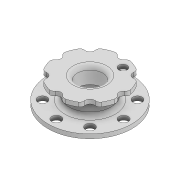
# Autodesk Inventor part: Pully_smlaller
Saved by Autodesk Inventor 2021 (Build 250183000, 183)
## iProperties
Created: 2022-09-22
Part Number: Pully_smlaller
Material: Generic
Document SubType Name: Modeling
Designer: ereg140
Density: 1 g/cm^3
Appearance: Default
Author: ereg140
Autodesk Inventor part; units mm, degrees
ref_plane "YZ Plane" through (0, 0, 0) normal (1, 0, 0) x (0, 1, 0)
ref_plane "XZ Plane" through (0, 0, 0) normal (0, 1, 0) x (-1, 0, 0)
ref_plane "XY Plane" through (0, 0, 0) normal (0, 0, 1) x (1, 0, 0)
sketch "Sketch1" plane through (0, 0, 0) normal (0, 1, 0) x (-1, 0, 0)
  circle A0 centre (0, 0) radius 12.0717
  line L0 (6, 10.475) -> (-6, 10.475)
  line L1 (9.5, 7.4482) -> (-9.5, 7.4482)
  dimension "d20" = 12
  dimension "d23" = 19
  dimension "d24" = 10.475
  constraints: 4 end point, 4 point on circle, 2 horizontal, 1 centre point, 1 coincident
  measures "d20" distance of L0.start L0.end
  measures "d23" distance of L1.start L1.end
  measures "d24" distance from line of point (0, 0) L0
extrude "Extrusion1" add sketch "Sketch1" along normal blind 3.8
sketch "Sketch2" plane through (0, 3.8, 0) normal (0, 1, 0) x (1, 0, 0)
  circle A0 centre (0, 0) radius 8 construction
  circle A1 centre (-8, 0) radius 1.1
  circle A2 centre (-5.6569, -5.6569) radius 1.1
  circle A3 centre (0, -8) radius 1.1
  circle A4 centre (5.6569, -5.6569) radius 1.1
  circle A5 centre (8, 0) radius 1.1
  circle A6 centre (5.6569, 5.6569) radius 1.1
  circle A7 centre (0, 8) radius 1.1
  circle A8 centre (-5.6569, 5.6569) radius 1.1
  circle A9 centre (0, 0) radius 5.5
  dimension "d3" = 16
  dimension "d4" = 2.2
  dimension "d7" = 360
  dimension "d9" = 11
  constraints: 9 centre point, 2 coincident, 2 horizontal alignment, 19 other
  measures "d4" diameter of A1
  measures "d9" diameter of A9
extrude "Extrusion2" cut sketch "Sketch2" against normal through all
sketch "Sketch3" plane through (0, 0, 0) normal (1, 0, 0) x (0, 1, 0)
  point P0 (0, 0)
sketch "Sketch4" plane through (0, 0, 0) normal (1, 0, 0) x (0, 1, 0)
  line L0 (3.8, 5.5) -> (0, 5.5) construction
  line L1 (0, 5.5) -> (0, 6.9) construction
  line L2 (0, 6.9) -> (3.8, 6.9) construction
  line L3 (3.8, 6.9) -> (3.8, 5.5) construction
  line L4 (0, -5.5) -> (3.8, -5.5) construction
  line L5 (3.8, -5.5) -> (3.8, -6.9) construction
  line L6 (3.8, -6.9) -> (0, -6.9) construction
  line L7 (0, -6.9) -> (0, -5.5) construction
  line L8 (0, 12.0717) -> (3.8, 12.0717) construction
  line L9 (3.8, 12.0717) -> (3.8, 9.1) construction
  line L10 (3.8, 9.1) -> (0, 9.1) construction
  line L11 (0, 9.1) -> (0, 12.0717) construction
  line L12 (3.8, -12.0717) -> (0, -12.0717) construction
  line L13 (0, -12.0717) -> (0, -9.1) construction
  line L14 (0, -9.1) -> (3.8, -9.1) construction
  line L15 (3.8, -9.1) -> (3.8, -12.0717) construction
  line L16 (0.6, -12.0717) -> (3.2, -12.0717)
  line L17 (3.2, -12.0717) -> (3.2, -9.5)
  line L18 (3.2, -9.5) -> (0.6, -9.5)
  line L19 (0.6, -9.5) -> (0.6, -12.0717)
  line L20 (-0.76, 0) -> (4.56, 0) projected
  point P0 (0, 0)
  point P1 (1.9, -12.0717)
  dimension "d12" = 0.6
  dimension "d15" = 9.5
  constraints: 8 end point, 2 midpoint, 2 parallel, 1 horizontal, 1 perpendicular
  measures "d12" distance between parallel lines of L13 L19
  measures "d15" distance from line of point (0, 0) L18
revolve "Revolution1" cut sketch "Sketch4" angle 360 about axis through (0, -10, 0) along (0, 1, 0)
sketch "Sketch5" plane through (0, 3.2, 0) normal (0, -1, 0) x (1, 0, 0)
  circle A0 centre (0, -10.1) radius 0.6
  circle A1 centre (0, 0) radius 9.5 construction
  circle A2 centre (0, 0) radius 12.0717 construction
  circle A3 centre (-8, 0) radius 1.1 construction
  circle A4 centre (8, 0) radius 1.1 construction
  circle A5 centre (5.6569, 5.6569) radius 1.1 construction
  circle A6 centre (-5.6569, -5.6569) radius 1.1 construction
  circle A7 centre (-5.6569, 5.6569) radius 1.1 construction
  circle A8 centre (5.6569, -5.6569) radius 1.1 construction
  circle A9 centre (0, 8) radius 1.1 construction
  circle A10 centre (0, -8) radius 1.1 construction
  circle A11 centre (0, 0) radius 5.5 construction
  dimension "d17" = 1.2
  constraints: 1 centre point, 1 tangent, 1 vertical alignment
  measures "d17" diameter of A0
extrude "Extrusion3" cut sketch "Sketch5" against normal up to surface (0.6 mm away)
sketch "Sketch6" plane through (0, 3.8, 0) normal (0, 1, 0) x (1, 0, 0)
  circle A0 centre (0, 0) radius 12.0717 projected
extrude "Extrusion4" cut sketch "Sketch6" against normal up to surface (3.2 mm away)
sketch "Sketch7" plane through (0, 0.6, 0) normal (0, 1, 0) x (1, 0, 0)
  circle A0 centre (0, 0) radius 5.5 projected
  circle A1 centre (0, 8) radius 1.1 projected
  circle A2 centre (0, -8) radius 1.1 projected
  circle A3 centre (5.6569, 5.6569) radius 1.1 projected
  circle A4 centre (-5.6569, -5.6569) radius 1.1 projected
  circle A5 centre (-5.6569, 5.6569) radius 1.1 projected
  circle A6 centre (5.6569, -5.6569) radius 1.1 projected
  circle A7 centre (8, 0) radius 1.1 projected
  circle A8 centre (-8, 0) radius 1.1 projected
  circle A9 centre (0, 0) radius 12.0717 projected
extrude "Extrusion5" add sketch "Sketch7" along normal blind 0.4
sketch "Sketch9" plane through (0, 0, 0) normal (0, -1, 0) x (1, 0, 0)
  circle A0 centre (0, 0) radius 4.25
  circle A1 centre (0, 0) radius 5.5 projected
  dimension "d29" = 8.5
  constraints: 1 centre point, 1 coincident
  measures "d29" diameter of A0
extrude "Extrusion6" add sketch "Sketch9" against normal up to surface (1 mm away)
sketch "Sketch10" plane through (0, 1, 0) normal (0, 1, 0) x (1, 0, 0)
  circle A0 centre (0, 0) radius 10
  circle A1 centre (0, 0) radius 12.0717 projected
  dimension "d32" = 20
  constraints: 1 centre point, 1 coincident
  measures "d32" diameter of A0
extrude "Extrusion7" cut sketch "Sketch10" against normal up to surface (1 mm away)
sketch "Sketch11" plane through (0, 1, 0) normal (0, 1, 0) x (1, 0, 0)
  circle A0 centre (0, 0) radius 5
  dimension "d35" = 10
  constraints: 1 centre point, 1 coincident
  measures "d35" diameter of A0
extrude "Extrusion8" add sketch "Sketch11" along normal blind 4
sketch "Sketch12" plane through (0, 1, 0) normal (0, -1, 0) x (1, 0, 0)
  circle A0 centre (0, 0) radius 4.25 projected
extrude "Extrusion9" cut sketch "Sketch12" against normal blind 1
sketch "Sketch13" plane through (0, 1, 0) normal (0, 1, 0) x (1, 0, 0)
  circle A0 centre (0, -8) radius 1.1 projected
  circle A1 centre (0, -8) radius 1.875
  point P0 (0, 0)
  dimension "d40" = 3.75
  constraints: 1 centre point, 1 coincident
  measures "d40" diameter of A1
fillet "Fillet1" radius 1 1 edges at (-5, 1, 0)
sketch "Sketch14" plane through (0, 5, 0) normal (0, 1, 0) x (1, 0, 0)
  circle A0 centre (0, -8) radius 1.1 projected
  circle A1 centre (0, 0) radius 8
  circle A2 centre (5.6569, -5.6569) radius 1.1 projected
  circle A3 centre (8, 0) radius 1.1 projected
  circle A4 centre (5.6569, 5.6569) radius 1.1 projected
  circle A5 centre (0, 8) radius 1.1 projected
  circle A6 centre (-5.6569, 5.6569) radius 1.1 projected
  circle A7 centre (-8, 0) radius 1.1 projected
  circle A8 centre (-5.6569, -5.6569) radius 1.1 projected
  point P0 (-6.3794, -4.8274)
  point P1 (-4.8274, -6.3794)
  point P2 (-1.0974, -7.9244)
  point P3 (1.0974, -7.9244)
  point P4 (4.8274, -6.3794)
  point P5 (6.3794, -4.8274)
  point P6 (7.9244, -1.0974)
  point P7 (7.9244, 1.0974)
  point P8 (6.3794, 4.8274)
  point P9 (4.8274, 6.3794)
  point P10 (1.0974, 7.9244)
  point P11 (-1.0974, 7.9244)
  point P12 (-4.8274, 6.3794)
  point P13 (-6.3794, 4.8274)
  point P14 (-7.9244, 1.0974)
  point P15 (-7.9244, -1.0974)
  constraints: 1 coincident, 3 other
extrude "Extrusion10" add sketch "Sketch14" along normal blind 1 contours A0 A1 A8 A7 A6 A5 A4 A3 A2
sketch "Sketch17" plane through (0, 6, 0) normal (0, 1, 0) x (1, 0, 0)
  circle A0 centre (0, 0) radius 3
  dimension "d49" = 6
  constraints: 1 centre point, 1 coincident
  measures "d49" diameter of A0
extrude "Extrusion12" cut sketch "Sketch17" against normal through all
fillet "Fillet3" radius 1 16 edges at (4.8274, 5.5, 6.3794) (6.3794, 5.5, 4.8274) (7.9244, 5.5, 1.0974) (7.9244, 5.5, -1.0974) (6.3794, 5.5, -4.8274) (4.8274, 5.5, -6.3794) (1.0974, 5.5, -7.9244) (-1.0974, 5.5, -7.9244) (-4.8274, 5.5, -6.3794) (-6.3794, 5.5, -4.8274) (-7.9244, 5.5, -1.0974) (-7.9244, 5.5, 1.0974) (-4.8274, 5.5, 6.3794) (-6.3794, 5.5, 4.8274) (-1.0974, 5.5, 7.9244) (1.0974, 5.5, 7.9244)
sketch "Sketch18" plane through (0, 6, 0) normal (0, 1, 0) x (1, 0, 0)
  circle A0 centre (0, 8) radius 1.1 construction
  circle A1 centre (5.6569, 5.6569) radius 1.1 construction
  line L0 (0, 0) -> (0, 8) construction
  line L1 (0, 0) -> (5.6569, 5.6569) construction
  line L2 (5.6569, 5.6569) -> (0, 8) construction
  line L3 (0, 0) -> (2.8284, 6.8284) construction
  circle A2 centre (2.2961, 5.5433) radius 1
  circle A3 centre (0, 0) radius 5 projected
  dimension "d53" = 2
  constraints: 8 end point, 1 centre point, 1 midpoint, 1 point on line, 1 tangent, 1 vertical
  measures "d53" diameter of A2
extrude "Extrusion13" cut sketch "Sketch18" against normal up to surface (1 mm away) contours A2
fillet "Fillet4" radius 1 1 edges at (-3, 6, 0)
fillet "Fillet5" radius 0.5 2 edges at (4.1573, 5, -2.7779) (-4.1573, 5, 2.7779)
body "Solid1"
